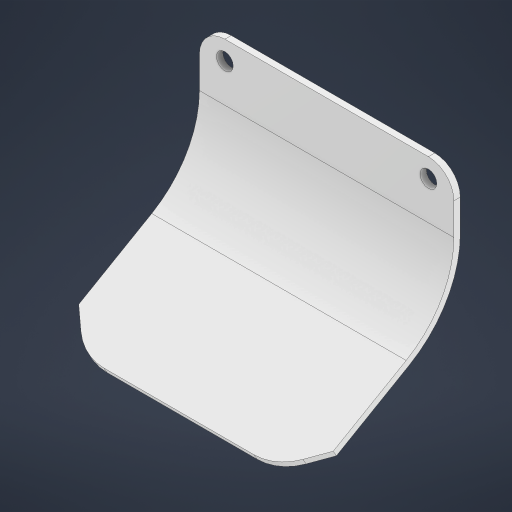
# Autodesk Inventor part: wedge
Saved by Autodesk Inventor 2024 (Build 280153000, 153)
## iProperties
Created: 2023-11-21
Part Number: wedge
Material: Acetal Resin, White
Document SubType Name: Sheet Metal
Designer: avere
Density: 1.425 g/cm^3
Appearance: Smooth - White
Flat Pattern Width: 6.87668 cm
Flat Pattern Length: 6.35 cm
Flat Pattern Area: 43.6669 cm^2
Sheet Metal Rule: Default
Sheet Metal Width: 2.707 in
Sheet Metal Length: 2.500 in
Sheet Metal Area: 6.768 in^2
Author: avere
Autodesk Inventor part; units mm, degrees
ref_plane "YZ Plane" through (0, 0, 0) normal (1, 0, 0) x (0, 1, 0)
ref_plane "XZ Plane" through (0, 0, 0) normal (0, 1, 0) x (-1, 0, 0)
ref_plane "XY Plane" through (0, 0, 0) normal (0, 0, 1) x (1, 0, 0)
sketch "Sketch1" plane through (0, 0, 0) normal (0, 0, 1) x (1, 0, 0)
  line L0 (-12.7, 4.7625) -> (38.1, 4.7625)
  line L1 (-15.875, -9.525) -> (44.45, -9.525)
  line L2 (-19.05, -1.5875) -> (-19.05, -26.8352)
  line L3 (44.45, -1.5875) -> (44.45, -30.4886)
  line L4 (-19.05, -9.525) -> (-15.875, -9.525)
  arc A0 (-12.7, 4.7625) -> (-19.05, -1.5875) centre (-12.7, -1.5875) ccw
  arc A1 (44.45, -1.5875) -> (38.1, 4.7625) centre (38.1, -1.5875) ccw
  line L5 (-19.05, -26.8352) -> (-19.05, -57.15)
  line L6 (-6.0043, -64.9352) -> (31.4043, -64.9352)
  line L7 (44.45, -57.15) -> (44.45, -30.4886)
  line L8 (-19.05, -57.15) -> (-14.9845, -61.2155)
  line L9 (-19.05, -57.15) -> (-13.3006, -57.15) construction
  line L10 (44.45, -57.15) -> (40.3845, -61.2155)
  line L11 (44.45, -57.15) -> (50.1994, -57.15) construction
  arc A2 (-14.9845, -61.2155) -> (-6.0043, -64.9352) centre (-6.0043, -52.2352) ccw
  arc A3 (31.4043, -64.9352) -> (40.3845, -61.2155) centre (31.4043, -52.2352) ccw
  circle A4 centre (-12.7, 0) radius 2.0955
  circle A5 centre (38.1, 0) radius 2.0955
  point P0 (0, 0)
  point P1 (25.4, 4.7625)
  point P2 (28.575, -33.6636)
  point P3 (-19.05, 4.7625)
  point P4 (44.45, 4.7625)
  point P5 (44.45, -30.1625)
  dimension "d10" = 6.35
  dimension "d13" = 45
  dimension "d14" = 135
  dimension "d15" = 12.7
  dimension "d16" = 4.191
  dimension "d17" = 4.191
  constraints: 24 end point, 8 point on circle, 8 point on line, 8 tangent, 6 centre point, 5 vertical, 3 horizontal, 2 equal length, 2 equal radius, 2 perpendicular, 1 collinear, 1 other
  measures "d10" radius of A0
  measures "d13" angle of L8 L9
  measures "d14" angle of L10 L11
  measures "d15" radius of A2
  measures "d16" diameter of A4
  measures "d17" diameter of A5
extrude "Extrusion1" add sketch "Sketch1" along normal blind 1.5875
bend part "Bend Part1" radius 25.4 angle 60 line through (-15.875, -9.525, 0) along (1, 0, 0) centre toward (0, 0, 1) moving side (0, -1, 0) both sides no
equation "\"BendRadius\" = Thickness"
equation "\"BendReliefWidth\" = Thickness"
equation "\"BendReliefDepth\" = 0.5 * Thickness"
equation "\"CornerReliefSize\" = 4 * Thickness"
equation "\"MinimumRemnant\" = 2 * Thickness"
equation "\"TransitionRadius\" = BendRadius"
equation "\"JacobiRadiusSize\" = BendRadius"
equation "\"GapSize\" = Thickness"
equation "\"Thickness\" = 1.5875"
body "Solid1"
